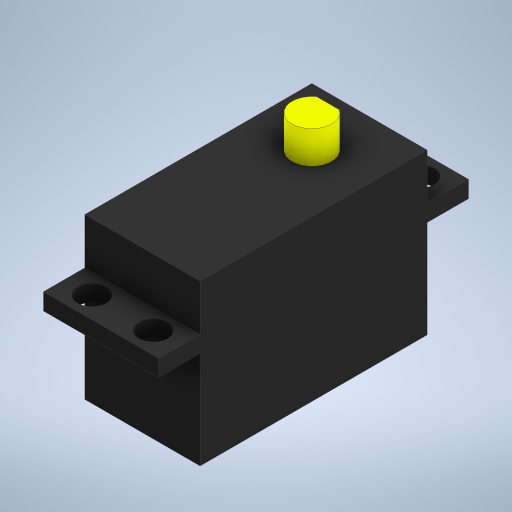
# Autodesk Inventor part: 감속기어 모터'
Saved by Autodesk Inventor 2023.1 (Build 271208000, 208)
## iProperties
Created: 2022-09-03
Part Number: 감속기어 모터'
Material: 일반
Document SubType Name: Modeling
Designer: fly01
Density: 1 g/cm^3
Appearance: 기본값
Author: fly01
Autodesk Inventor part; units mm, degrees
ref_plane "YZ Plane" through (0, 0, 0) normal (1, 0, 0) x (0, 1, 0)
ref_plane "XZ Plane" through (0, 0, 0) normal (0, 1, 0) x (-1, 0, 0)
ref_plane "XY Plane" through (0, 0, 0) normal (0, 0, 1) x (1, 0, 0)
sketch "스케치1" plane through (0, 0, 0) normal (0, 1, 0) x (-1, 0, 0)
  line L0 (-8, 15.75) -> (8, 15.75)
  line L1 (8, 15.75) -> (8, -15.75)
  line L2 (8, -15.75) -> (-8, -15.75)
  line L3 (-8, -15.75) -> (-8, 15.75)
  line L4 (-8, 15.75) -> (8, -15.75) construction
  line L5 (8, 15.75) -> (-8, -15.75) construction
  point P0 (0, 0)
  dimension "d0" = 16
  dimension "d1" = 31.5
  constraints: 12 end point, 2 midpoint, 2 parallel, 1 horizontal, 1 perpendicular
  measures "d0" distance of L1.end L2.end
  measures "d1" distance of L0.end L1.end
extrude "돌출1" add sketch "스케치1" along normal blind 13.5
sketch "스케치2" plane through (0, 13.5, 0) normal (0, 1, 0) x (1, 0, 0)
  line L0 (-8, -21.5) -> (8, -21.5)
  line L1 (8, -21.5) -> (8, 21.5)
  line L2 (8, 21.5) -> (-8, 21.5)
  line L3 (-8, 21.5) -> (-8, -21.5)
  line L4 (-8, -21.5) -> (8, 21.5) construction
  line L5 (8, -21.5) -> (-8, 21.5) construction
  circle A0 centre (-4.25, -18.5) radius 2
  line L6 (0, 0) -> (0, -2.2737)
  line L7 (0, 0) -> (-1.7913, 0)
  circle A1 centre (4.25, -18.5) radius 2
  circle A2 centre (-4.25, 18.5) radius 2
  circle A3 centre (4.25, 18.5) radius 2
  point P0 (-8, 15.75)
  dimension "d4" = 43
  dimension "d5" = 4
  dimension "d6" = 37
  dimension "d7" = 8.5
  constraints: 16 end point, 4 centre point, 3 symmetric about line, 2 horizontal, 2 midpoint, 2 parallel, 1 perpendicular, 1 point on line, 1 vertical, 3 other
  measures "d4" distance of L2.end L0.start
  measures "d5" diameter of A0
  measures "d6" distance of A2.centre A0.centre
  measures "d7" distance of A1.centre A0.centre
extrude "돌출2" add sketch "스케치2" along normal blind 2.3
extrude "돌출3" add sketch "스케치1" along normal blind 22.2
sketch "스케치4" plane through (0, 22.2, 0) normal (0, 1, 0) x (1, 0, 0)
  circle A0 centre (0, 7.75) radius 2.75
  line L0 (8, 15.75) -> (-8, 15.75) projected
  line L1 (-1.5811, 10) -> (1.5811, 10)
  point P0 (0, 0)
  dimension "d12" = 8
  dimension "d13" = 5.5
  dimension "d14" = 0.5
  constraints: 2 end point, 2 point on circle, 1 centre point, 1 horizontal
  measures "d12" distance from line of L0 A0.centre
  measures "d13" diameter of A0
  measures "d14" distance edge to line of A0 L1
extrude "돌출4" add sketch "스케치4" along normal blind 4.5 contours A0 L1 picked at (-0.1073, 8.3396)
